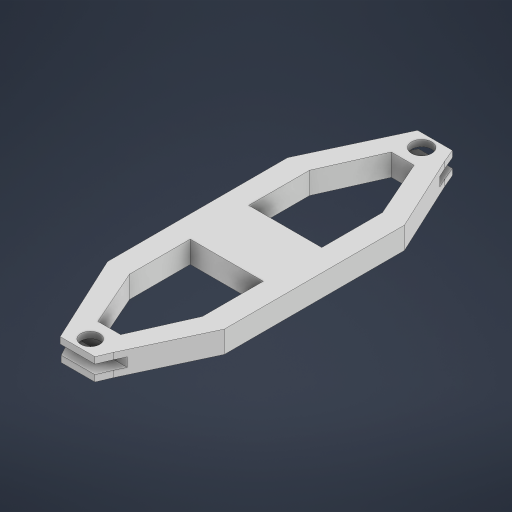
# Autodesk Inventor part: Diff_BarV2
Saved by Autodesk Inventor 2023 (Build 270158000, 158)
## iProperties
Created: 2023-04-06
Part Number: Diff_BarV2
Material: Generic
Document SubType Name: Modeling
Designer: bugme
Density: 1 g/cm^3
Appearance: Default
Author: bugme
Autodesk Inventor part; units mm, degrees
ref_plane "YZ Plane" through (0, 0, 0) normal (1, 0, 0) x (0, 1, 0)
ref_plane "XZ Plane" through (0, 0, 0) normal (0, 1, 0) x (-1, 0, 0)
ref_plane "XY Plane" through (0, 0, 0) normal (0, 0, 1) x (1, 0, 0)
sketch "Sketch1" plane through (0, 0, 0) normal (0, 1, 0) x (-1, 0, 0)
  line L0 (0, -213.8682) -> (0, 213.8682) projected
  line L1 (20.1057, -144) -> (-20.1057, -144)
  line L2 (-50.827, -78.2337) -> (-50.827, 78.2337)
  line L3 (-20.1057, 144) -> (20.1057, 144)
  line L4 (50.773, 78.2337) -> (50.773, -78.2337)
  line L5 (158.1712, 0) -> (-85.66, 0) projected
  line L6 (50.773, 78.2337) -> (20.1057, 144)
  line L7 (50.773, 78.2337) -> (123.3381, 78.2337) construction
  line L8 (-50.827, 78.2337) -> (-20.1057, 144)
  line L9 (-20.1057, 144) -> (20.1057, 144)
  line L10 (31.723, 78.2337) -> (31.723, -78.2337)
  line L11 (-31.777, -78.2337) -> (-31.777, 78.2337)
  line L12 (-20.1057, -144) -> (20.1057, -144)
  line L13 (50.773, -78.2337) -> (20.1057, -144)
  line L14 (-50.827, -78.2337) -> (-20.1057, -144)
  line L15 (31.723, -25.4) -> (31.723, 25.4)
  line L16 (31.723, -25.4) -> (-31.777, -25.4)
  line L17 (31.723, 25.4) -> (-31.777, 25.4)
  line L18 (31.723, 78.2337) -> (9.9071, 127.5128)
  line L19 (-31.777, 78.2337) -> (-9.9611, 127.5128)
  line L20 (-9.9611, 127.5128) -> (9.9071, 127.5128)
  line L21 (50.773, 78.2337) -> (31.723, 78.2337)
  line L22 (-31.777, 78.2337) -> (-50.827, 78.2337)
  line L23 (31.723, -78.2337) -> (9.9071, -127.5128)
  line L24 (-31.777, -78.2337) -> (-9.9611, -127.5128)
  line L25 (-9.9611, -127.5128) -> (9.9071, -127.5128)
  line L26 (50.773, -78.2337) -> (31.723, -78.2337)
  line L27 (-31.777, -78.2337) -> (-50.827, -78.2337)
  point P0 (50.8, -140)
  point P1 (-50.8, 140)
  point P2 (-50.8, -140)
  dimension "d49" = 280
  dimension "d51" = 115
  dimension "d52" = 101.6
  dimension "d53" = 50.8
  dimension "d71" = 288
  constraints: 52 end point, 10 symmetric about line, 7 horizontal, 4 point on line, 3 parallel, 2 perpendicular, 1 equal length
  measures "d49" distance of point (-50.8, -140) point (-50.8, 140)
  measures "d51" angle of L7 L6
  measures "d52" distance between parallel lines of L2 L4
  measures "d53" distance of L15.start L15.end
  measures "d71" distance between parallel lines of L1 L3
extrude "Extrusion1" add sketch "Sketch1" along normal blind 19.05 contours L1 L14 L27 L24 L25 L0 | L0 L25 L23 L26 L13 L1 | L16 L11 L5 L0 | L0 L5 L10 L16 | L26 L10 L5 L4 | L2 L5 L11 L27 | L5 L11 L17 L0 | L0 L17 L10 L5 | L5 L10 L21 L4 | L2 L22 L11 L5 | L21 L18 L20 L0 L3 L6 | L8 L3 L0 L20 L19 L22
sketch "Sketch9" plane through (50.827, 0, 78.2337) normal (1, 0, 0) x (0, 0, -1)
  line L0 (-65.7663, 19.05) -> (0, 19.05) projected
  line L1 (-65.7663, 19.05) -> (-65.7663, 0)
  line L2 (-65.7663, 0) -> (-65.7663, 19.05) projected
  line L3 (-65.7663, 9.525) -> (-52.4585, 9.525)
  line L4 (-65.7663, 13.4938) -> (-65.7663, 5.5563)
  line L5 (-65.7663, 19.05) -> (-77.0693, 19.05)
  line L6 (-65.7663, 19.05) -> (-54.4633, 19.05) construction
  line L7 (-65.7663, 13.4938) -> (-77.0693, 13.4937)
  line L8 (-77.0693, 13.4937) -> (-77.0693, 19.05)
  line L9 (-65.7663, 19.05) -> (-65.7663, 13.4938)
  line L10 (78.2337, -3.81) -> (78.2337, 22.86) projected
  line L11 (222.2337, 19.05) -> (233.5367, 19.05)
  line L12 (222.2337, 13.4938) -> (233.5367, 13.4937)
  line L13 (233.5367, 13.4937) -> (233.5367, 19.05)
  line L14 (222.2337, 19.05) -> (222.2337, 13.4938)
  point P0 (78.2337, 0)
  dimension "d55" = 7.9375
  dimension "d56" = 11.303
  dimension "d57" = 180
  constraints: 24 end point, 5 symmetric about line, 4 horizontal, 2 collinear, 2 point on line, 1 midpoint, 1 perpendicular, 1 vertical
  measures "d55" distance of L4.start L4.end
  measures "d56" distance of L0.start L5.end
  measures "d57" angle of L5 L6
extrude "Extrusion9" add sketch "Sketch9" against normal up to surface (70.9326 mm away)
sketch "Sketch10" plane through (0, 19.05, 0) normal (0, 1, 0) x (1, 0, 0)
  line L0 (20.1057, -144) -> (50.827, -78.2337) projected
  line L1 (20.1057, -144) -> (15.3607, -155.303)
  line L2 (50.827, -155.303) -> (-20.1057, -155.303) projected
  line L3 (15.3607, -155.303) -> (50.53, -155.303)
  line L4 (50.827, -144) -> (20.1057, -144) projected
  line L5 (20.1057, -144) -> (50.827, -144)
  line L6 (50.827, -144) -> (50.827, -155.303) projected
  line L7 (50.827, -144) -> (50.827, -155.303)
  line L8 (50.827, -155.303) -> (50.827, -144)
  line L9 (50.827, -155.303) -> (15.3607, -155.303)
  line L10 (-71.093, 0) -> (71.147, 0) projected
  line L11 (20.1057, 144) -> (15.3607, 155.303)
  line L12 (15.3607, 155.303) -> (50.53, 155.303)
  line L13 (50.827, 144) -> (20.1057, 144)
  line L14 (20.1057, 144) -> (50.827, 144)
  line L15 (50.827, 144) -> (50.827, 155.303)
  line L16 (50.827, 144) -> (50.827, 155.303)
  line L17 (50.827, 155.303) -> (50.827, 144)
  line L18 (50.827, 155.303) -> (15.3607, 155.303)
  line L19 (-20.1057, -144) -> (-14.8343, -155.303)
  line L20 (-20.1057, -155.303) -> (-14.8343, -155.303)
  line L21 (-50.773, -78.2337) -> (-20.1057, -144) projected
  line L22 (-20.1057, -155.303) -> (-20.1057, -144)
  line L23 (-20.1057, 144) -> (-14.8343, 155.303)
  line L24 (-20.1057, 155.303) -> (-14.8343, 155.303)
  line L25 (-20.1057, 155.303) -> (-20.1057, 144)
  point P0 (0, 0)
  constraints: 40 end point, 8 symmetric about line, 2 collinear, 2 horizontal, 2 perpendicular, 1 midpoint, 1 point on line
extrude "Extrusion10" cut sketch "Sketch10" against normal up to surface (19.05 mm away)
sketch "Sketch11" plane through (50.827, 0, 78.2337) normal (1, 0, 0) x (0, 0, -1)
  line L0 (-65.7663, 0) -> (-65.7663, 13.4938) projected
  line L1 (-65.7663, 0) -> (-77.0693, 0)
  line L2 (-77.0693, 0) -> (-77.0693, 5.5626)
  line L3 (-77.0693, 5.5626) -> (-65.7663, 5.5626)
  line L4 (-77.0693, 19.05) -> (-65.7663, 19.05) projected
  line L5 (78.2337, -3.81) -> (78.2337, 22.86) projected
  line L6 (222.2337, 0) -> (233.5367, 0)
  line L7 (233.5367, 0) -> (233.5367, 5.5626)
  line L8 (233.5367, 5.5626) -> (222.2337, 5.5626)
  line L9 (222.2337, 0) -> (222.2337, 13.4938) projected
  line L10 (222.2337, 5.5626) -> (222.2337, 0)
  point P0 (78.2337, 0)
  dimension "d63" = 5.5626
  dimension "d76" = 11.303
  constraints: 14 end point, 4 symmetric about line, 2 vertical, 1 horizontal, 1 perpendicular, 1 point on line
  measures "d63" distance of L1.end L2.end
  measures "d76" distance of L2.end L3.end
extrude "Extrusion11" add sketch "Sketch11" against normal up to surface (70.9326 mm away)
sketch "Sketch12" plane through (50.827, 5.5626, -144) normal (0, 1, 0) x (1, 0, 0)
  line L0 (-70.9326, 11.303) -> (-70.9326, 0) projected
  line L1 (-70.9326, 11.303) -> (-70.9326, 0)
  line L2 (-70.9326, 0) -> (-64.7758, 11.303)
  line L3 (-64.7758, 11.303) -> (-70.9326, 11.303)
  line L4 (-35.4663, 11.303) -> (-65.6612, 11.303) projected
  line L5 (-35.4663, 11.303) -> (-30.7213, 0)
  line L6 (0, 0) -> (0, 11.303) projected
  line L7 (-30.7213, 0) -> (0, 0)
  line L8 (0, 0) -> (0, 11.303)
  line L9 (0, 11.303) -> (-35.4663, 11.303)
  line L10 (-121.92, -144) -> (20.32, -144) projected
  line L11 (-70.9326, -299.303) -> (-70.9326, -288)
  line L12 (-70.9326, -299.303) -> (-70.9326, -288)
  line L13 (-70.9326, -288) -> (-64.7758, -299.303)
  line L14 (-64.7758, -299.303) -> (-70.9326, -299.303)
  line L15 (-35.4663, -299.303) -> (-65.6612, -299.303)
  line L16 (-35.4663, -299.303) -> (-30.7213, -288)
  line L17 (0, -288) -> (0, -299.303)
  line L18 (-30.7213, -288) -> (0, -288)
  line L19 (0, -288) -> (0, -299.303)
  line L20 (0, -299.303) -> (-35.4663, -299.303)
  point P0 (-50.827, -144)
  constraints: 34 end point, 8 symmetric about line, 3 perpendicular, 2 collinear
extrude "Extrusion12" cut sketch "Sketch12" against normal through all
sketch "Sketch13" plane through (0, 19.05, 0) normal (0, 1, 0) x (1, 0, 0)
  circle A0 centre (0, -144) radius 8.1915
  circle A1 centre (0, 144) radius 8.763
  line L0 (-71.093, 0) -> (71.147, 0) projected
  point P0 (0, 0)
  dimension "d68" = 16.383
  dimension "d69" = 17.526
  dimension "d70" = 288
  constraints: 2 centre point, 1 symmetric about line
  measures "d68" diameter of A0
  measures "d69" diameter of A1
  measures "d70" distance of A1.centre A0.centre
extrude "Extrusion13" cut sketch "Sketch13" against normal up to surface (13.4874 mm away)
sketch "Sketch14" plane through (50.827, 0, 78.2337) normal (1, 0, 0) x (0, 0, -1)
  line L0 (-57.5748, 19.05) -> (-57.5748, 5.5626) projected
  line L1 (-57.5748, 19.05) -> (-57.5748, 5.5626) projected
  line L2 (-57.5748, 19.05) -> (-57.5748, 5.5626) projected
  line L3 (-65.7663, 13.4938) -> (-57.5748, 13.4938)
  line L4 (-57.5748, 5.5626) -> (-57.5748, 13.4938)
  line L5 (-65.7663, 5.5626) -> (-65.7663, 13.4938) projected
  line L6 (-57.5748, 5.5626) -> (-65.7663, 5.5626)
  line L7 (78.2337, -3.81) -> (78.2337, 22.86) projected
  line L8 (222.2337, 13.4938) -> (214.0422, 13.4938)
  line L9 (214.0422, 5.5626) -> (214.0422, 13.4938)
  line L10 (222.2337, 5.5626) -> (222.2337, 13.4938)
  line L11 (214.0422, 5.5626) -> (222.2337, 5.5626)
  point P0 (78.2337, 0)
  constraints: 14 end point, 6 symmetric about line, 1 collinear, 1 horizontal, 1 point on line
extrude "Extrusion14" cut sketch "Sketch14" against normal through all
body "Solid1"
